Autodesk Inventor part; units mm, degrees
(part 3 of 3)
ref_plane "to_Bolt_1_56_ZX" through (-118.4211, 0, -250) normal (0, 0, -1) x (0, 1, 0)
ref_plane "to_Bolt_1_57_XY" through (-116.0287, 0, -250) normal (0, 1, 0) x (1, 0, 0)
ref_plane "to_Bolt_1_57_YZ" through (-116.0287, 0, -250) normal (1, 0, 0) x (0, 0, -1)
ref_plane "to_Bolt_1_57_ZX" through (-116.0287, 0, -250) normal (0, 0, -1) x (0, 1, 0)
ref_plane "to_Bolt_1_58_XY" through (-113.6364, 0, -250) normal (0, 1, 0) x (1, 0, 0)
ref_plane "to_Bolt_1_58_YZ" through (-113.6364, 0, -250) normal (1, 0, 0) x (0, 0, -1)
ref_plane "to_Bolt_1_58_ZX" through (-113.6364, 0, -250) normal (0, 0, -1) x (0, 1, 0)
ref_plane "to_Bolt_1_59_XY" through (-111.244, 0, -250) normal (0, 1, 0) x (1, 0, 0)
ref_plane "to_Bolt_1_59_YZ" through (-111.244, 0, -250) normal (1, 0, 0) x (0, 0, -1)
ref_plane "to_Bolt_1_59_ZX" through (-111.244, 0, -250) normal (0, 0, -1) x (0, 1, 0)
ref_plane "to_Bolt_1_6_XY" through (-238.0383, 0, -250) normal (0, 1, 0) x (1, 0, 0)
ref_plane "to_Bolt_1_6_YZ" through (-238.0383, 0, -250) normal (1, 0, 0) x (0, 0, -1)
ref_plane "to_Bolt_1_6_ZX" through (-238.0383, 0, -250) normal (0, 0, -1) x (0, 1, 0)
ref_plane "to_Bolt_1_60_XY" through (-108.8517, 0, -250) normal (0, 1, 0) x (1, 0, 0)
ref_plane "to_Bolt_1_60_YZ" through (-108.8517, 0, -250) normal (1, 0, 0) x (0, 0, -1)
ref_plane "to_Bolt_1_60_ZX" through (-108.8517, 0, -250) normal (0, 0, -1) x (0, 1, 0)
ref_plane "to_Bolt_1_61_XY" through (-106.4593, 0, -250) normal (0, 1, 0) x (1, 0, 0)
ref_plane "to_Bolt_1_61_YZ" through (-106.4593, 0, -250) normal (1, 0, 0) x (0, 0, -1)
ref_plane "to_Bolt_1_61_ZX" through (-106.4593, 0, -250) normal (0, 0, -1) x (0, 1, 0)
ref_plane "to_Bolt_1_62_XY" through (-104.067, 0, -250) normal (0, 1, 0) x (1, 0, 0)
ref_plane "to_Bolt_1_62_YZ" through (-104.067, 0, -250) normal (1, 0, 0) x (0, 0, -1)
ref_plane "to_Bolt_1_62_ZX" through (-104.067, 0, -250) normal (0, 0, -1) x (0, 1, 0)
ref_plane "to_Bolt_1_63_XY" through (-101.6746, 0, -250) normal (0, 1, 0) x (1, 0, 0)
ref_plane "to_Bolt_1_63_YZ" through (-101.6746, 0, -250) normal (1, 0, 0) x (0, 0, -1)
ref_plane "to_Bolt_1_63_ZX" through (-101.6746, 0, -250) normal (0, 0, -1) x (0, 1, 0)
ref_plane "to_Bolt_1_64_XY" through (-99.2823, 0, -250) normal (0, 1, 0) x (1, 0, 0)
ref_plane "to_Bolt_1_64_YZ" through (-99.2823, 0, -250) normal (1, 0, 0) x (0, 0, -1)
ref_plane "to_Bolt_1_64_ZX" through (-99.2823, 0, -250) normal (0, 0, -1) x (0, 1, 0)
ref_plane "to_Bolt_1_65_XY" through (-96.89, 0, -250) normal (0, 1, 0) x (1, 0, 0)
ref_plane "to_Bolt_1_65_YZ" through (-96.89, 0, -250) normal (1, 0, 0) x (0, 0, -1)
ref_plane "to_Bolt_1_65_ZX" through (-96.89, 0, -250) normal (0, 0, -1) x (0, 1, 0)
ref_plane "to_Bolt_1_66_XY" through (-94.4976, 0, -250) normal (0, 1, 0) x (1, 0, 0)
ref_plane "to_Bolt_1_66_YZ" through (-94.4976, 0, -250) normal (1, 0, 0) x (0, 0, -1)
ref_plane "to_Bolt_1_66_ZX" through (-94.4976, 0, -250) normal (0, 0, -1) x (0, 1, 0)
ref_plane "to_Bolt_1_67_XY" through (-92.1053, 0, -250) normal (0, 1, 0) x (1, 0, 0)
ref_plane "to_Bolt_1_67_YZ" through (-92.1053, 0, -250) normal (1, 0, 0) x (0, 0, -1)
ref_plane "to_Bolt_1_67_ZX" through (-92.1053, 0, -250) normal (0, 0, -1) x (0, 1, 0)
ref_plane "to_Bolt_1_68_XY" through (-89.7129, 0, -250) normal (0, 1, 0) x (1, 0, 0)
ref_plane "to_Bolt_1_68_YZ" through (-89.7129, 0, -250) normal (1, 0, 0) x (0, 0, -1)
ref_plane "to_Bolt_1_68_ZX" through (-89.7129, 0, -250) normal (0, 0, -1) x (0, 1, 0)
ref_plane "to_Bolt_1_69_XY" through (-87.3206, 0, -250) normal (0, 1, 0) x (1, 0, 0)
ref_plane "to_Bolt_1_69_YZ" through (-87.3206, 0, -250) normal (1, 0, 0) x (0, 0, -1)
ref_plane "to_Bolt_1_69_ZX" through (-87.3206, 0, -250) normal (0, 0, -1) x (0, 1, 0)
ref_plane "to_Bolt_1_7_XY" through (-235.6459, 0, -250) normal (0, 1, 0) x (1, 0, 0)
ref_plane "to_Bolt_1_7_YZ" through (-235.6459, 0, -250) normal (1, 0, 0) x (0, 0, -1)
ref_plane "to_Bolt_1_7_ZX" through (-235.6459, 0, -250) normal (0, 0, -1) x (0, 1, 0)
ref_plane "to_Bolt_1_70_XY" through (-84.9282, 0, -250) normal (0, 1, 0) x (1, 0, 0)
ref_plane "to_Bolt_1_70_YZ" through (-84.9282, 0, -250) normal (1, 0, 0) x (0, 0, -1)
ref_plane "to_Bolt_1_70_ZX" through (-84.9282, 0, -250) normal (0, 0, -1) x (0, 1, 0)
ref_plane "to_Bolt_1_71_XY" through (-82.5359, 0, -250) normal (0, 1, 0) x (1, 0, 0)
ref_plane "to_Bolt_1_71_YZ" through (-82.5359, 0, -250) normal (1, 0, 0) x (0, 0, -1)
ref_plane "to_Bolt_1_71_ZX" through (-82.5359, 0, -250) normal (0, 0, -1) x (0, 1, 0)
ref_plane "to_Bolt_1_72_XY" through (-80.1435, 0, -250) normal (0, 1, 0) x (1, 0, 0)
ref_plane "to_Bolt_1_72_YZ" through (-80.1435, 0, -250) normal (1, 0, 0) x (0, 0, -1)
ref_plane "to_Bolt_1_72_ZX" through (-80.1435, 0, -250) normal (0, 0, -1) x (0, 1, 0)
ref_plane "to_Bolt_1_73_XY" through (-77.7512, 0, -250) normal (0, 1, 0) x (1, 0, 0)
ref_plane "to_Bolt_1_73_YZ" through (-77.7512, 0, -250) normal (1, 0, 0) x (0, 0, -1)
ref_plane "to_Bolt_1_73_ZX" through (-77.7512, 0, -250) normal (0, 0, -1) x (0, 1, 0)
ref_plane "to_Bolt_1_74_XY" through (-75.3589, 0, -250) normal (0, 1, 0) x (1, 0, 0)
ref_plane "to_Bolt_1_74_YZ" through (-75.3589, 0, -250) normal (1, 0, 0) x (0, 0, -1)
ref_plane "to_Bolt_1_74_ZX" through (-75.3589, 0, -250) normal (0, 0, -1) x (0, 1, 0)
ref_plane "to_Bolt_1_75_XY" through (-72.9665, 0, -250) normal (0, 1, 0) x (1, 0, 0)
ref_plane "to_Bolt_1_75_YZ" through (-72.9665, 0, -250) normal (1, 0, 0) x (0, 0, -1)
ref_plane "to_Bolt_1_75_ZX" through (-72.9665, 0, -250) normal (0, 0, -1) x (0, 1, 0)
ref_plane "to_Bolt_1_76_XY" through (-70.5742, 0, -250) normal (0, 1, 0) x (1, 0, 0)
ref_plane "to_Bolt_1_76_YZ" through (-70.5742, 0, -250) normal (1, 0, 0) x (0, 0, -1)
ref_plane "to_Bolt_1_76_ZX" through (-70.5742, 0, -250) normal (0, 0, -1) x (0, 1, 0)
ref_plane "to_Bolt_1_77_XY" through (-68.1818, 0, -250) normal (0, 1, 0) x (1, 0, 0)
ref_plane "to_Bolt_1_77_YZ" through (-68.1818, 0, -250) normal (1, 0, 0) x (0, 0, -1)
ref_plane "to_Bolt_1_77_ZX" through (-68.1818, 0, -250) normal (0, 0, -1) x (0, 1, 0)
ref_plane "to_Bolt_1_78_XY" through (-65.7895, 0, -250) normal (0, 1, 0) x (1, 0, 0)
ref_plane "to_Bolt_1_78_YZ" through (-65.7895, 0, -250) normal (1, 0, 0) x (0, 0, -1)
ref_plane "to_Bolt_1_78_ZX" through (-65.7895, 0, -250) normal (0, 0, -1) x (0, 1, 0)
ref_plane "to_Bolt_1_79_XY" through (-63.3971, 0, -250) normal (0, 1, 0) x (1, 0, 0)
ref_plane "to_Bolt_1_79_YZ" through (-63.3971, 0, -250) normal (1, 0, 0) x (0, 0, -1)
ref_plane "to_Bolt_1_79_ZX" through (-63.3971, 0, -250) normal (0, 0, -1) x (0, 1, 0)
ref_plane "to_Bolt_1_8_XY" through (-233.2536, 0, -250) normal (0, 1, 0) x (1, 0, 0)
ref_plane "to_Bolt_1_8_YZ" through (-233.2536, 0, -250) normal (1, 0, 0) x (0, 0, -1)
ref_plane "to_Bolt_1_8_ZX" through (-233.2536, 0, -250) normal (0, 0, -1) x (0, 1, 0)
ref_plane "to_Bolt_1_80_XY" through (-61.0048, 0, -250) normal (0, 1, 0) x (1, 0, 0)
ref_plane "to_Bolt_1_80_YZ" through (-61.0048, 0, -250) normal (1, 0, 0) x (0, 0, -1)
ref_plane "to_Bolt_1_80_ZX" through (-61.0048, 0, -250) normal (0, 0, -1) x (0, 1, 0)
ref_plane "to_Bolt_1_81_XY" through (-58.6124, 0, -250) normal (0, 1, 0) x (1, 0, 0)
ref_plane "to_Bolt_1_81_YZ" through (-58.6124, 0, -250) normal (1, 0, 0) x (0, 0, -1)
ref_plane "to_Bolt_1_81_ZX" through (-58.6124, 0, -250) normal (0, 0, -1) x (0, 1, 0)
ref_plane "to_Bolt_1_82_XY" through (-56.2201, 0, -250) normal (0, 1, 0) x (1, 0, 0)
ref_plane "to_Bolt_1_82_YZ" through (-56.2201, 0, -250) normal (1, 0, 0) x (0, 0, -1)
ref_plane "to_Bolt_1_82_ZX" through (-56.2201, 0, -250) normal (0, 0, -1) x (0, 1, 0)
ref_plane "to_Bolt_1_83_XY" through (-53.8278, 0, -250) normal (0, 1, 0) x (1, 0, 0)
ref_plane "to_Bolt_1_83_YZ" through (-53.8278, 0, -250) normal (1, 0, 0) x (0, 0, -1)
ref_plane "to_Bolt_1_83_ZX" through (-53.8278, 0, -250) normal (0, 0, -1) x (0, 1, 0)
ref_plane "to_Bolt_1_84_XY" through (-51.4354, 0, -250) normal (0, 1, 0) x (1, 0, 0)
ref_plane "to_Bolt_1_84_YZ" through (-51.4354, 0, -250) normal (1, 0, 0) x (0, 0, -1)
ref_plane "to_Bolt_1_84_ZX" through (-51.4354, 0, -250) normal (0, 0, -1) x (0, 1, 0)
ref_plane "to_Bolt_1_85_XY" through (-49.0431, 0, -250) normal (0, 1, 0) x (1, 0, 0)
ref_plane "to_Bolt_1_85_YZ" through (-49.0431, 0, -250) normal (1, 0, 0) x (0, 0, -1)
ref_plane "to_Bolt_1_85_ZX" through (-49.0431, 0, -250) normal (0, 0, -1) x (0, 1, 0)
ref_plane "to_Bolt_1_86_XY" through (-46.6507, 0, -250) normal (0, 1, 0) x (1, 0, 0)
ref_plane "to_Bolt_1_86_YZ" through (-46.6507, 0, -250) normal (1, 0, 0) x (0, 0, -1)
ref_plane "to_Bolt_1_86_ZX" through (-46.6507, 0, -250) normal (0, 0, -1) x (0, 1, 0)
ref_plane "to_Bolt_1_87_XY" through (-44.2584, 0, -250) normal (0, 1, 0) x (1, 0, 0)
ref_plane "to_Bolt_1_87_YZ" through (-44.2584, 0, -250) normal (1, 0, 0) x (0, 0, -1)
ref_plane "to_Bolt_1_87_ZX" through (-44.2584, 0, -250) normal (0, 0, -1) x (0, 1, 0)
ref_plane "to_Bolt_1_88_XY" through (-41.866, 0, -250) normal (0, 1, 0) x (1, 0, 0)
ref_plane "to_Bolt_1_88_YZ" through (-41.866, 0, -250) normal (1, 0, 0) x (0, 0, -1)
ref_plane "to_Bolt_1_88_ZX" through (-41.866, 0, -250) normal (0, 0, -1) x (0, 1, 0)
ref_plane "to_Bolt_1_89_XY" through (-39.4737, 0, -250) normal (0, 1, 0) x (1, 0, 0)
ref_plane "to_Bolt_1_89_YZ" through (-39.4737, 0, -250) normal (1, 0, 0) x (0, 0, -1)
ref_plane "to_Bolt_1_89_ZX" through (-39.4737, 0, -250) normal (0, 0, -1) x (0, 1, 0)
ref_plane "to_Bolt_1_9_XY" through (-230.8612, 0, -250) normal (0, 1, 0) x (1, 0, 0)
ref_plane "to_Bolt_1_9_YZ" through (-230.8612, 0, -250) normal (1, 0, 0) x (0, 0, -1)
ref_plane "to_Bolt_1_9_ZX" through (-230.8612, 0, -250) normal (0, 0, -1) x (0, 1, 0)
ref_plane "to_Bolt_1_90_XY" through (-37.0813, 0, -250) normal (0, 1, 0) x (1, 0, 0)
ref_plane "to_Bolt_1_90_YZ" through (-37.0813, 0, -250) normal (1, 0, 0) x (0, 0, -1)
ref_plane "to_Bolt_1_90_ZX" through (-37.0813, 0, -250) normal (0, 0, -1) x (0, 1, 0)
ref_plane "to_Bolt_1_91_XY" through (-34.689, 0, -250) normal (0, 1, 0) x (1, 0, 0)
ref_plane "to_Bolt_1_91_YZ" through (-34.689, 0, -250) normal (1, 0, 0) x (0, 0, -1)
ref_plane "to_Bolt_1_91_ZX" through (-34.689, 0, -250) normal (0, 0, -1) x (0, 1, 0)
ref_plane "to_Bolt_1_92_XY" through (-32.2967, 0, -250) normal (0, 1, 0) x (1, 0, 0)
ref_plane "to_Bolt_1_92_YZ" through (-32.2967, 0, -250) normal (1, 0, 0) x (0, 0, -1)
ref_plane "to_Bolt_1_92_ZX" through (-32.2967, 0, -250) normal (0, 0, -1) x (0, 1, 0)
ref_plane "to_Bolt_1_93_XY" through (-29.9043, 0, -250) normal (0, 1, 0) x (1, 0, 0)
ref_plane "to_Bolt_1_93_YZ" through (-29.9043, 0, -250) normal (1, 0, 0) x (0, 0, -1)
ref_plane "to_Bolt_1_93_ZX" through (-29.9043, 0, -250) normal (0, 0, -1) x (0, 1, 0)
ref_plane "to_Bolt_1_94_XY" through (-27.512, 0, -250) normal (0, 1, 0) x (1, 0, 0)
ref_plane "to_Bolt_1_94_YZ" through (-27.512, 0, -250) normal (1, 0, 0) x (0, 0, -1)
ref_plane "to_Bolt_1_94_ZX" through (-27.512, 0, -250) normal (0, 0, -1) x (0, 1, 0)
ref_plane "to_Bolt_1_95_XY" through (-25.1196, 0, -250) normal (0, 1, 0) x (1, 0, 0)
ref_plane "to_Bolt_1_95_YZ" through (-25.1196, 0, -250) normal (1, 0, 0) x (0, 0, -1)
ref_plane "to_Bolt_1_95_ZX" through (-25.1196, 0, -250) normal (0, 0, -1) x (0, 1, 0)
ref_plane "to_Bolt_1_96_XY" through (-22.7273, 0, -250) normal (0, 1, 0) x (1, 0, 0)
ref_plane "to_Bolt_1_96_YZ" through (-22.7273, 0, -250) normal (1, 0, 0) x (0, 0, -1)
ref_plane "to_Bolt_1_96_ZX" through (-22.7273, 0, -250) normal (0, 0, -1) x (0, 1, 0)
ref_plane "to_Bolt_1_97_XY" through (-20.3349, 0, -250) normal (0, 1, 0) x (1, 0, 0)
ref_plane "to_Bolt_1_97_YZ" through (-20.3349, 0, -250) normal (1, 0, 0) x (0, 0, -1)
ref_plane "to_Bolt_1_97_ZX" through (-20.3349, 0, -250) normal (0, 0, -1) x (0, 1, 0)
ref_plane "to_Bolt_1_98_XY" through (-17.9426, 0, -250) normal (0, 1, 0) x (1, 0, 0)
ref_plane "to_Bolt_1_98_YZ" through (-17.9426, 0, -250) normal (1, 0, 0) x (0, 0, -1)
ref_plane "to_Bolt_1_98_ZX" through (-17.9426, 0, -250) normal (0, 0, -1) x (0, 1, 0)
ref_plane "to_Bolt_1_99_XY" through (-15.5502, 0, -250) normal (0, 1, 0) x (1, 0, 0)
ref_plane "to_Bolt_1_99_YZ" through (-15.5502, 0, -250) normal (1, 0, 0) x (0, 0, -1)
ref_plane "to_Bolt_1_99_ZX" through (-15.5502, 0, -250) normal (0, 0, -1) x (0, 1, 0)
ref_plane "to_Bolt_2_XY" through (250, 0, -250) normal (0, 1, 0) x (1, 0, 0)
ref_plane "to_Bolt_2_YZ" through (250, 0, -250) normal (1, 0, 0) x (0, 0, -1)
ref_plane "to_Bolt_2_ZX" through (250, 0, -250) normal (0, 0, -1) x (0, 1, 0)
ref_plane "to_Bolt_3_XY" through (-250, 0, 250) normal (0, 1, 0) x (1, 0, 0)
ref_plane "to_Bolt_3_YZ" through (-250, 0, 250) normal (1, 0, 0) x (0, 0, -1)
ref_plane "to_Bolt_3_ZX" through (-250, 0, 250) normal (0, 0, -1) x (0, 1, 0)
ref_plane "to_Bolt_4_XY" through (250, 0, 250) normal (0, 1, 0) x (1, 0, 0)
ref_plane "to_Bolt_4_YZ" through (250, 0, 250) normal (1, 0, 0) x (0, 0, -1)
ref_plane "to_Bolt_4_ZX" through (250, 0, 250) normal (0, 0, -1) x (0, 1, 0)
body "Solid1"
